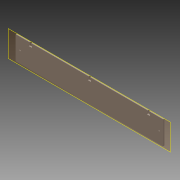
# Autodesk Inventor part: Panel_front
Saved by Autodesk Inventor 2013 (Build 170138000, 138)
## iProperties
Created: 2013-02-02
Part Number: Panel_front
Material: Aluminum 6061
Document SubType Name: Modeling
Designer: xylzlyx
Density: 1 g/cm^3
Author: xylzlyx
Autodesk Inventor part; units mm, degrees
ref_plane "YZ Plane" through (0, 0, 0) normal (1, 0, 0) x (0, 1, 0)
ref_plane "XZ Plane" through (0, 0, 0) normal (0, 1, 0) x (-1, 0, 0)
ref_plane "XY Plane" through (0, 0, 0) normal (0, 0, 1) x (1, 0, 0)
ref_plane "Work Plane1" through (0, 0, -9.525) normal (0, 0, 1) x (1, 0, 0)
sketch "Sketch1" plane through (0, 0, -9.525) normal (0, 0, 1) x (1, 0, 0)
  line L0 (381, -60.8043) -> (381, -64.0283) construction
  line L1 (381, -64.0283) -> (0, -64.0283) construction
  line L2 (0, -64.0283) -> (0, -60.8043) construction
  line L3 (0, -60.8043) -> (381, -60.8043) construction
  line L4 (381, 0) -> (0, 0) construction
  line L5 (0, 0) -> (0, 3.175) construction
  line L6 (0, 3.175) -> (381, 3.175) construction
  line L7 (381, 3.175) -> (381, 0) construction
  line L8 (381, -60.8043) -> (0, -60.8043)
  line L9 (0, -60.8043) -> (0, 0)
  line L10 (0, 0) -> (381, 0)
  line L11 (381, 0) -> (381, -60.8043)
  constraints: 24 end point, 5 horizontal, 4 coincident, 4 vertical, 2 parallel, 1 perpendicular, 8 other
extrude "FrontPanel" add sketch "Sketch1" against normal blind 3.175
fillet "CornerFillet" radius 1 4 edges at (381, -60.8043, -11.1125) (0, -60.8043, -11.1125) (0, 0, -11.1125) (381, 0, -11.1125)
sketch "ScrewSlotSketch" plane through (0, 0, -9.525) normal (0, 0, 1) x (1, 0, 0)
  line L0 (368.3, -28.0035) -> (368.3, -1) projected
  line L1 (12.7, -1) -> (12.7, -28.0035) projected
  line L2 (381, 0) -> (0, 0) construction
  line L3 (0, 0) -> (0, 3.175) construction
  line L4 (0, 3.175) -> (381, 3.175) construction
  line L5 (381, 3.175) -> (381, 0) construction
  line L6 (381, -60.8043) -> (381, -64.0283) construction
  line L7 (381, -64.0283) -> (0, -64.0283) construction
  line L8 (0, -64.0283) -> (0, -60.8043) construction
  line L9 (0, -60.8043) -> (381, -60.8043) construction
  line L10 (344.7987, -9.525) -> (344.7987, 3.175)
  line L11 (344.7987, 3.175) -> (341.0014, 3.175)
  line L12 (341.0014, 3.175) -> (341.0014, -9.525)
  line L13 (341.0014, -9.525) -> (344.7987, -9.525)
  line L14 (346.9958, -9.525) -> (338.8043, -9.525)
  line L15 (338.8043, -9.525) -> (338.8043, -6.4929)
  line L16 (338.8043, -6.4929) -> (346.9958, -6.4929)
  line L17 (346.9958, -6.4929) -> (346.9958, -9.525)
  line L18 (36.2014, -9.525) -> (39.9987, -9.525)
  line L19 (39.9987, -9.525) -> (39.9987, 3.175)
  line L20 (39.9987, 3.175) -> (36.2014, 3.175)
  line L21 (36.2014, 3.175) -> (36.2014, -9.525)
  line L22 (34.0043, -9.525) -> (42.1958, -9.525)
  line L23 (42.1958, -9.525) -> (42.1958, -6.4929)
  line L24 (42.1958, -6.4929) -> (34.0043, -6.4929)
  line L25 (34.0043, -6.4929) -> (34.0043, -9.525)
  line L26 (192.3987, -9.525) -> (188.6014, -9.525)
  line L27 (188.6014, -9.525) -> (188.6014, 3.175)
  line L28 (188.6014, 3.175) -> (192.3987, 3.175)
  line L29 (192.3987, 3.175) -> (192.3987, -9.525)
  line L30 (186.4043, -9.525) -> (194.5958, -9.525)
  line L31 (194.5958, -9.525) -> (194.5958, -6.4929)
  line L32 (194.5958, -6.4929) -> (186.4043, -6.4929)
  line L33 (186.4043, -6.4929) -> (186.4043, -9.525)
  point P0 (342.9, 3.175)
  point P1 (342.9, -9.525)
  point P2 (38.1, -9.525)
  point P3 (38.1, 3.175)
  point P4 (190.5, -9.525)
  point P5 (190.5, 3.175)
  dimension "d4" = 12.7
  dimension "d6" = 3.7973
  dimension "d7" = 25.4
  dimension "d8" = 8.1915
  dimension "d9" = 3.0321
  dimension "d10" = 3.7973
  dimension "d11" = 12.7
  dimension "d12" = 8.1915
  dimension "d13" = 3.0321
  dimension "d14" = 25.4
  dimension "d15" = 3.7973
  dimension "d16" = 12.7
  dimension "d17" = 3.0321
  dimension "d18" = 8.1915
  constraints: 64 end point, 15 parallel, 10 midpoint, 8 horizontal, 4 perpendicular, 4 vertical, 2 point on line, 1 collinear, 7 other
  measures "d4" distance of L10.start L10.end
  measures "d6" distance of L10.end L11.end
  measures "d7" distance from line of L0 point (342.9, 3.175)
  measures "d8" distance of L14.start L14.end
  measures "d9" distance of L14.end L15.end
  measures "d10" distance of L19.end L20.end
  measures "d11" distance of L20.end L18.start
  measures "d12" distance of L22.start L22.end
  measures "d13" distance of L22.end L23.end
  measures "d14" distance from line of L1 point (38.1, 3.175)
  measures "d15" distance of L27.end L28.end
  measures "d16" distance of L26.end L27.end
  measures "d17" distance of L32.end L30.start
  measures "d18" distance of L30.start L30.end
extrude "ScrewSlotExtrusion" cut sketch "ScrewSlotSketch" against normal blind 3.175
fillet "ScrewSlotFillet" radius 0.5 24 edges at (344.7987, 0, -11.1125) (341.0014, 0, -11.1125) (344.7987, -6.4929, -11.1125) (341.0014, -6.4929, -11.1125) (338.8043, -6.4929, -11.1125) (338.8043, -9.525, -11.1125) (346.9958, -9.525, -11.1125) (346.9958, -6.4929, -11.1125) (192.3987, 0, -11.1125) (188.6014, 0, -11.1125) (192.3987, -6.4929, -11.1125) (188.6014, -6.4929, -11.1125) (194.5958, -6.4929, -11.1125) (194.5958, -9.525, -11.1125) (186.4043, -6.4929, -11.1125) (186.4043, -9.525, -11.1125) (42.1958, -9.525, -11.1125) (42.1958, -6.4929, -11.1125) (39.9987, -6.4929, -11.1125) (39.9987, 0, -11.1125) (36.2014, 0, -11.1125) (36.2014, -6.4929, -11.1125) (34.0043, -6.4929, -11.1125) (34.0043, -9.525, -11.1125)
sketch "ScrewHoleSketch" plane through (0, 0, -9.525) normal (0, 0, 1) x (1, 0, 0)
  line L0 (34.0043, -9.025) -> (34.0043, -6.9929) projected
  line L1 (368.3, -28.5035) -> (371.475, -28.5035) projected
  line L2 (371.475, -32.3008) -> (368.3, -32.3008) projected
  line L3 (9.525, -28.5035) -> (12.7, -28.5035) projected
  line L4 (12.7, -32.3008) -> (9.525, -32.3008) projected
  line L5 (371.475, -28.5035) -> (371.475, -32.3008) construction
  line L6 (9.525, -28.5035) -> (9.525, -32.3008) construction
  point P0 (0, 0)
  point P1 (11.1125, -30.4021)
  point P2 (369.8875, -30.4021)
  point P3 (369.8875, -28.5035)
  point P4 (371.475, -30.4021)
  point P5 (9.525, -30.4021)
  point P6 (11.1125, -28.5035)
  constraints: 4 end point, 4 midpoint, 2 horizontal alignment, 2 parallel, 2 vertical alignment
hole "ScrewHoles" at (11.1125, -30.4021, -9.525) at (369.8875, -30.4021, -9.525) direction (0, 0, -1) diameter 3.7973 end through all
equation "\"d4\" = ScrewLen"
equation "\"d6\" = ScrewHoleD"
equation "\"d7\" = ScrewHoleDist"
equation "\"d8\" = NutFlatsGap"
equation "\"d9\" = NutHeightGap"
equation "\"d10\" = ScrewHoleD"
equation "\"d11\" = ScrewLen"
equation "\"d12\" = NutFlatsGap"
equation "\"d13\" = NutHeightGap"
equation "\"d14\" = ScrewHoleDist"
equation "\"d15\" = ScrewHoleD"
equation "\"d16\" = ScrewLen"
equation "\"d17\" = NutHeightGap"
equation "\"d18\" = NutFlatsGap"
equation "\"d21\" = SlotFilletRad"
equation "\"d22\" = ScrewHoleD"
equation "\"ScrewLen\" = 12.7"
equation "\"ScrewHoleD\" = 3.7973"
equation "\"NutFlatsGap\" = 8.1915"
equation "\"NutHeightGap\" = 3.032125"
equation "\"SlotFilletRad\" = 0.5"
equation "\"ScrewHoleDist\" = 25.4"
body "Solid1"
